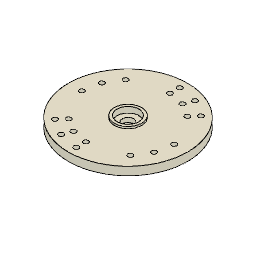
FT90R (Assembly) (Autodesk Fusion 360 archive; units mm, degrees)
design "Disc Servo Attachment"
Autodesk Fusion 360 part; units mm, degrees
sketch "Sketch1" plane through (0, 0, 0) normal (0, 1, 0) x (1, 0, 0)
  circle A0 centre (0, 0) radius 3.4163
  circle A1 centre (0, 0) radius 2.3241
  dimension "d1" = 6.8326
  dimension "d2" = 4.6482
  constraint coincident A0.centre A1.centre
  constraint concentric A0 A1
  measures "d1" diameter of A0
  measures "d2" diameter of A1
extrude "Extrude1" add sketch "Sketch1" along normal blind 2.3368 makes body 1
sketch "Sketch2" plane through (0, 2.3368, 0) normal (0, 1, 0) x (-1, 0, 0)
  circle A0 centre (0, 0) radius 2.3241
  circle A1 centre (0, 0) radius 3.4163
  circle A2 centre (0, 0) radius 11.8872
  circle A3 centre (0, 0) radius 1.1303
  dimension "d5" = 23.7744
  dimension "d6" = 2.2606
  constraint coincident A0.centre A1.centre
  constraint concentric A2 A3
  measures "d5" diameter of A2
  measures "d6" diameter of A3
extrude "Extrude2" add sketch "Sketch2" along normal blind 1.651 separate body contours A0 | A1 | A2 makes body 2
sketch "Sketch3" plane through (0, 3.9878, 0) normal (0, 1, 0) x (-1, 0, 0)
  circle A0 centre (0, 0) radius 1.1303
  circle A1 centre (0, 0) radius 11.8872
  circle A2 centre (0, 0) radius 2.7178
  circle A3 centre (0, 0) radius 2.1844
  dimension "d9" = 5.4356
  dimension "d10" = 4.3688
  constraint concentric A0 A2
  constraint coincident A0.centre A1.centre
  measures "d9" diameter of A2
  measures "d10" diameter of A3
extrude "Extrude3" add sketch "Sketch3" along normal blind 0.381 contours A2 bodies 2
sketch "Sketch4" plane through (0, 3.9878, 0) normal (0, 1, 0) x (-1, 0, 0)
  circle A0 centre (0, 0) radius 11.8872
  circle A1 centre (0, 0) radius 2.7178
  circle A2 centre (0, 0) radius 10.2872 construction
  circle A3 centre (0, 0) radius 9.2202 construction
  circle A4 centre (0, 0) radius 8.382 construction
  line L0 (0, 2.7178) -> (0, -10.795) construction
  circle A5 centre (-0.0124, -10.2872) radius 0.508
  circle A6 centre (0, -8.382) radius 0.508
  circle A7 centre (0, 0) radius 11.8872 construction
  line L1 (0, -10.795) -> (0, -11.8872) construction
  line L2 (0, -11.8872) -> (0, -8.89) construction
  circle A8 centre (-3.0695, -7.7998) radius 0.508
  circle A9 centre (-3.7556, -9.5771) radius 0.508
  circle A10 centre (-5.6936, -6.1515) radius 0.508
  circle A11 centre (-6.9837, -7.5534) radius 0.508
  line L3 (0.4991, -8.4767) -> (-3.5686, -7.7051) construction
  line L4 (0.4867, -10.3818) -> (-4.2547, -9.4824) construction
  line L5 (-2.6393, -8.07) -> (-6.1237, -5.8813) construction
  line L6 (-3.3252, -9.8469) -> (-7.4141, -7.2835) construction
  line L7 (0, 0) -> (-11.8872, 0) construction
  circle A12 centre (-9.2202, 0) radius 0.508
  line L8 (-11.8872, 0) -> (-9.7282, 0) construction
  circle A13 centre (-8.5826, 3.3692) radius 0.508
  circle A14 centre (-6.7579, 6.2724) radius 0.508
  line L9 (-9.3147, -0.4991) -> (-8.4881, 3.8683) construction
  line L10 (-8.8529, 2.9391) -> (-6.4876, 6.7025) construction
  circle A15 centre (0.0124, 10.2872) radius 0.508
  circle A16 centre (0, 8.382) radius 0.508
  circle A17 centre (3.7556, 9.5771) radius 0.508
  circle A18 centre (3.0695, 7.7998) radius 0.508
  circle A19 centre (6.9837, 7.5534) radius 0.508
  circle A20 centre (5.6936, 6.1515) radius 0.508
  circle A21 centre (9.2202, 0) radius 0.508
  circle A22 centre (8.5826, -3.3692) radius 0.508
  circle A23 centre (6.7579, -6.2724) radius 0.508
  dimension "d13" = 1.016
  dimension "d14" = 1.016
  dimension "d16" = 1.0922
  dimension "d17" = 2.9972
  dimension "d18" = 1.016
  dimension "d19" = 1.016
  dimension "d20" = 1.016
  dimension "d21" = 1.016
  dimension "d22" = 4.1402
  dimension "d23" = 4.826
  dimension "d24" = 4.1148
  dimension "d25" = 4.826
  dimension "d26" = 1.016
  dimension "d27" = 2.159
  dimension "d28" = 1.016
  dimension "d29" = 1.016
  dimension "d30" = 4.445
  dimension "d31" = 4.445
  dimension "d32" = 1.016
  dimension "d33" = 1.016
  dimension "d34" = 1.016
  dimension "d35" = 1.016
  dimension "d36" = 1.016
  dimension "d37" = 1.016
  dimension "d38" = 1.016
  dimension "d39" = 1.016
  dimension "d40" = 1.016
  constraint concentric A0 A2
  constraint concentric A0 A3
  constraint coincident A0.centre A1.centre
  constraint vertical L0
  constraint coincident A4 A6.centre
  constraint coincident L0 A6.centre
  constraint coincident A1 L0.start
  constraint concentric A4 A7
  constraint equal A0 A7
  constraint coincident A5 L0.end
  constraint coincident A7 L1.end
  constraint parallel L0 L1
  constraint coincident L0 L2.end
  constraint coincident A6 L2.end
  constraint coincident A2 A5.centre
  constraint coincident A4 A8.centre
  constraint coincident A2 A9.centre
  constraint coincident A4 A10.centre
  constraint coincident A2 A11.centre
  constraint coincident A6 L3.start
  constraint coincident A8 L3.end
  constraint coincident A5 L4.start
  constraint coincident A9 L4.end
  constraint parallel L3 L4
  constraint coincident A6.centre L3
  constraint coincident A8.centre L3
  constraint coincident A5.centre L4
  constraint coincident A9.centre L4
  constraint coincident A8 L5.start
  constraint coincident A10 L5.end
  constraint coincident A9 L6.start
  constraint coincident A11 L6.end
  constraint coincident A8.centre L5
  constraint coincident A10.centre L5
  constraint coincident A9.centre L6
  constraint coincident A11.centre L6
  constraint coincident A7 L7.end
  constraint perpendicular L0 L7
  constraint coincident A3 A12.centre
  constraint coincident L7 A12.centre
  constraint coincident A12 L8.end
  constraint coincident L7 L8.end
  constraint coincident A3 A13.centre
  constraint coincident A3 A14.centre
  constraint coincident A12 L9.start
  constraint coincident A13 L9.end
  constraint coincident A13 L10.start
  constraint coincident A14 L10.end
  constraint coincident A12.centre L9
  constraint coincident A13.centre L9
  constraint coincident A13.centre L10
  constraint coincident A14.centre L10
  constraint coincident A0.centre L0
  measures "d13" diameter of A5
  measures "d14" diameter of A6
  measures "d16" distance of L0.end L1.end
  measures "d17" distance of L1.end L2.end
  measures "d18" diameter of A8
  measures "d19" diameter of A9
  measures "d20" diameter of A10
  measures "d21" diameter of A11
  measures "d22" distance of L3.start L3.end
  measures "d23" distance of L4.start L4.end
  measures "d24" distance of L5.start L5.end
  measures "d25" distance of L6.start L6.end
  measures "d26" diameter of A12
  measures "d27" distance of L7.end L8.end
  measures "d28" diameter of A13
  measures "d29" diameter of A14
  measures "d30" distance of L9.start L9.end
  measures "d31" distance of L10.start L10.end
  measures "d32" diameter of A15
  measures "d33" diameter of A16
  measures "d34" diameter of A18
  measures "d35" diameter of A17
  measures "d36" diameter of A20
  measures "d37" diameter of A19
  measures "d38" diameter of A21
  measures "d39" diameter of A22
  measures "d40" diameter of A23
hole "Hole1" at (0.0124, 3.9878, -10.2872) at (0, 3.9878, -8.382) at (3.7556, 3.9878, -9.5771) at (3.0695, 3.9878, -7.7998) at (6.9837, 3.9878, -7.5534) at (5.6936, 3.9878, -6.1515) at (9.2202, 3.9878, 0) at (8.5826, 3.9878, 3.3692) at (6.7579, 3.9878, 6.2724) at (-0.0124, 3.9878, 10.2872) at (0, 3.9878, 8.382) at (-3.0695, 3.9878, 7.7998) at (-3.7556, 3.9878, 9.5771) at (-6.9837, 3.9878, 7.5534) at (-5.6936, 3.9878, 6.1515) at (-9.2202, 3.9878, 0) at (-8.5826, 3.9878, -3.3692) at (-6.7579, 3.9878, -6.2724) direction (0, -1, 0) diameter 1 end through all bodies 2
extrude "Extrude4" cut 1 faces at (-1.8207, 3.9878, -0.1647) along direction (0, -1, 0) blind 1.143 from surface at -0.381 on bodies 2 bodies 2

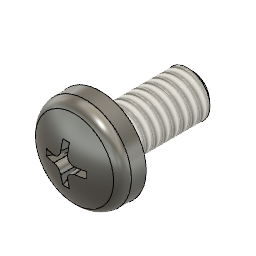
design "Pan Head Screw UNI EN ISO 7045 - M2 x 4 - H Steel 4.6 Plain"
description: Pan Head Screw UNI EN ISO 7045 - M2 x 4 - H
part number: UNI EN ISO 7045 - M2 x 4 - H Steel 4.6 Plain
Autodesk Fusion 360 part; units mm, degrees
sketch "Sketch1" plane through (0, 0, 0) normal (0, 1, 0) x (1, 0, 0)
  line L0 (-1, 0.8) -> (-1, 4)
  line L1 (-1, 4) -> (0, 4)
  line L2 (0, 4) -> (0, -1.6)
  line L3 (-0.8917, 0) -> (-2, 0)
  arc A0 (-1.9678, -0.9235) -> (0, -1.6) centre (0, 1.6) ccw
  line L4 (-1, 0.8) -> (-0.8917, 0.5678)
  line L5 (-0.8917, 0.5678) -> (-0.8917, 0)
  line L6 (-2, 0) -> (-1.9678, -0.9235)
  dimension "d9" = 2
  dimension "d66" = 4
  dimension "d75" = 1.7835
  dimension "d77" = 0.8
  dimension "d78" = 155
  dimension "d103" = 2
  dimension "d111" = 1.6
  dimension "d112" = 4
  constraint perpendicular L0 L1
  constraint collinear origin L2.end L1.end
  constraint perpendicular L0 L3
  constraint coincident origin L3
  constraint vertical L0
  constraint vertical L2
  constraint coincident L2 A0.centre
  constraint perpendicular L3 L5
  constraint coincident L3.start L5.end
  measures "d77" distance of L3 L0.start
  measures "d78" angle of L0 L4
  measures "d103" angle of L2 L6
  measures "d111" distance of L2.end L3
  measures "d112" distance of origin L1
revolve "Revolve1" add sketch "Sketch1" angle 360 about axis through (0, 0, -4) along (0, 0, 1) makes body 1
ref_plane "WorkPlane1" through (0, 0, 1.6) normal (0, 0, 1) x (1, 0, 0)
sketch "Sketch2" plane through (0, 0, 1.6) normal (0, 0, 1) x (1, 0, 0)
  line L0 (-0.15, 0.15) -> (-0.95, 0.15)
  line L1 (-0.15, -0.15) -> (-0.95, -0.15)
  line L2 (-0.95, 0.15) -> (-0.95, -0.15)
  line L3 (-0.15, -0.15) -> (-0.15, -0.95)
  line L4 (-0.15, -0.95) -> (0.15, -0.95)
  line L5 (0.15, -0.15) -> (0.15, -0.95)
  line L6 (0.15, -0.15) -> (0.95, -0.15)
  line L7 (0.95, -0.15) -> (0.95, 0.15)
  line L8 (0.15, 0.15) -> (0.95, 0.15)
  line L9 (0.15, 0.15) -> (0.15, 0.95)
  line L10 (0.15, 0.95) -> (-0.15, 0.95)
  line L11 (-0.15, 0.15) -> (-0.15, 0.95)
  dimension "d105" = 0.3
  dimension "d107" = 360
  dimension "d108" = 1.9
  constraint perpendicular L1 L2
  constraint vertical L0.start L1.start
  constraint horizontal L1
  constraint coincident L8.start L9.start
  measures "d105" distance of L0 L1
  measures "d108" distance of L2 L7
extrude "Extrude1" add sketch "Sketch2" against normal blind 1.2 draft -4 separate body makes body 2
draft "Draft1" angle -30 neutral plane through (0, 0, 1.6) pull (0, 0, 1) 4 faces at (-0.922, -0.022, 1.2) (-0.022, -0.922, 1.2) (0.922, -0.022, 1.2) (0.022, 0.922, 1.2) on bodies 2
fillet "Fillet3" radius 0.3 4 edges at (0.108, 0.108, 1) (-0.108, 0.108, 1) (0.108, -0.108, 1) (-0.108, -0.108, 1) on bodies 2
combine "Combine1" operation cut target body 1 tool bodies 2
fillet "Fillet4" radius 0.6 1 edges at (-1.8346, 0.7116, 0.9235) on bodies 1
thread "Thread1" "ISO Metric profile 2.0 M2x0.4 M2x0.4 6g" major diameter 1.9335 minor diameter 1.478 pitch 0.4 angle 60 resizes the face on face at (-0.9988, 0.0498, -1.8667) on bodies 1
fillet "Fillet5" radius 0.2 1 edges at (-0.8314, 0.3225, 0) on bodies 1
sketch "Sketch5" plane through (0, 0, 0) normal (0, 1, 0) x (1, 0, 0)
  line L0 (-1.02, 4) -> (-1.02, 3.7546)
  line L1 (-1.02, 3.7546) -> (-0.7546, 4)
  line L2 (0, 4) -> (0, -1.6)
  line L3 (-1.02, 4) -> (0, 4)
  dimension "d114" = 0.2454
  dimension "d115" = 1.02
  dimension "d116" = 0.2654
  constraint coincident L2.start L3.end
  constraint perpendicular L2 L3
  constraint coincident L1.end L3
  constraint perpendicular L0 L3
  measures "d114" distance of L0.end L3
  measures "d115" distance of L0 L2.start
  measures "d116" distance of L0 L1.end
revolve "Revolve2" cut sketch "Sketch5" angle 360 about axis through (0, 0, -4) along (0, 0, 1) bodies 1
equation "d9 = adsk_nomdia"
equation "adsk_nomlen = 4.00 mm"
equation "adsk_headh = 1.60 mm"
equation "adsk_headdia = 4.00 mm"
equation "adsk_nomdia = 2.00 mm"
equation "adsk_phildia = 1.90 mm"
equation "d31 = -adsk_phildepth"
equation "adsk_philwidth = 0.30 mm"
equation "adsk_phildepth = 1.20 mm"
equation "d66 = adsk_headdia"
equation "d71 = adsk_headh"
equation "adsk_thrlen = 3.20 mm"
equation "d75 = adsk_shnkdia"
equation "adsk_shnkdia = 1.78349 mm"
equation "d77 = adsk_nomlen - adsk_thrlen"
equation "adsk_endpointdia = 1.50924 mm"
equation "adsk_startlen = 0.24538 mm"
equation "adsk_ovalrad = 3.20 mm"
equation "adsk_headtoprad = adsk_nomdia * 0.3"
equation "adsk_midfillet = adsk_nomdia * 0.1"
equation "d98 = adsk_midfillet"
equation "adsk_headang = 2.00 deg"
equation "d102 = adsk_headtoprad"
equation "d103 = adsk_headang"
equation "d105 = adsk_philwidth"
equation "d108 = adsk_phildia"
equation "d110 = adsk_philwidth"
equation "d111 = adsk_headh"
equation "d112 = adsk_nomlen"
equation "d113 = ( adsk_nomlen + adsk_headh ) - ( adsk_ovalrad )"
equation "d114 = adsk_startlen"
equation "d115 = adsk_nomdia * 0.51"
equation "d116 = ( adsk_nomdia * 0.51 ) - ( adsk_endpointdia / 2 )"

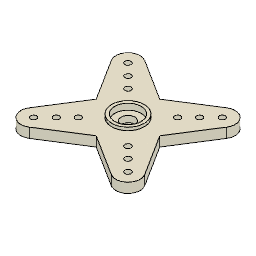
design "Square Servo Attachment"
Autodesk Fusion 360 part; units mm, degrees
sketch "Sketch1" plane through (0, 0, 0) normal (0, 1, 0) x (1, 0, 0)
  circle A0 centre (0, 0) radius 3.3909
  circle A1 centre (0, 0) radius 2.3368
  dimension "d1" = 6.7818
  dimension "d2" = 4.6736
  constraint coincident A0.centre A1.centre
  measures "d1" diameter of A0
  measures "d2" diameter of A1
extrude "Extrude1" add sketch "Sketch1" along normal blind 1.9304
sketch "Sketch2" plane through (0, 1.9304, 0) normal (0, 1, 0) x (-1, 0, 0)
  circle A0 centre (0, 0) radius 2.3368
  circle A1 centre (0, 0) radius 3.3909
  line L0 (-10.0076, 10.0076) -> (10.0076, 10.0076) construction
  line L1 (10.0076, 10.0076) -> (10.0076, -10.0076) construction
  line L2 (10.0076, -10.0076) -> (-10.0076, -10.0076) construction
  line L3 (-10.0076, -10.0076) -> (-10.0076, 10.0076) construction
  line L4 (-10.0076, 10.0076) -> (10.0076, -10.0076) construction
  line L5 (10.0076, 10.0076) -> (-10.0076, -10.0076) construction
  circle A2 centre (7.9709, -7.9709) radius 2.0367 construction
  circle A3 centre (-7.9709, -7.9709) radius 2.0367 construction
  circle A4 centre (-7.9709, 7.9709) radius 2.0367 construction
  circle A5 centre (7.9709, 7.9709) radius 2.0367 construction
  circle A6 centre (0, 0) radius 5.334 construction
  circle A7 centre (7.9709, -7.9709) radius 0.5
  circle A8 centre (-7.9709, -7.9709) radius 0.5
  circle A9 centre (7.9709, 7.9709) radius 0.5
  circle A10 centre (-7.9709, 7.9709) radius 0.5
  line L6 (8.4709, -7.9709) -> (-8.4709, -7.9709) construction
  line L7 (0, -5.334) -> (0, 5.334) construction
  line L8 (5.334, 0) -> (-5.334, 0) construction
  line L9 (9.4111, -6.5307) -> (6.5307, -9.4111) construction
  line L10 (-6.5307, -9.4111) -> (-9.4111, -6.5307) construction
  line L11 (-9.4111, 6.5307) -> (-6.5307, 9.4111) construction
  line L12 (9.4111, 6.5307) -> (6.5307, 9.4111) construction
  line L13 (5.334, 0) -> (9.6916, -6.8813)
  line L14 (5.334, 0) -> (9.6916, 6.8813)
  line L15 (0, 5.334) -> (6.8813, 9.6916)
  line L16 (0, 5.334) -> (-6.8813, 9.6916)
  line L17 (-5.334, 0) -> (-9.6916, 6.8813)
  line L18 (-5.334, 0) -> (-9.6916, -6.8813)
  line L19 (0, -5.334) -> (-6.8813, -9.6916)
  line L20 (0, -5.334) -> (6.8813, -9.6916)
  arc A11 (6.8813, -9.6916) -> (9.6916, -6.8813) centre (7.9709, -7.9709) ccw
  arc A12 (-9.6916, -6.8813) -> (-6.8813, -9.6916) centre (-7.9709, -7.9709) ccw
  arc A13 (-6.8813, 9.6916) -> (-9.6916, 6.8813) centre (-7.9709, 7.9709) ccw
  arc A14 (9.6916, 6.8813) -> (6.8813, 9.6916) centre (7.9709, 7.9709) ccw
  circle A15 centre (0, 0) radius 1.143
  dimension "d5" = 20.0152
  dimension "d6" = 20.0152
  dimension "d7" = 10.668
  dimension "d8" = 1
  dimension "d9" = 16.9418
  dimension "d10" = 2.286
  constraint horizontal L0
  constraint perpendicular L0 L1
  constraint parallel L0 L2
  constraint parallel L1 L3
  constraint coincident L4 A0.centre
  constraint coincident L5 A0.centre
  constraint coincident A0.centre A1.centre
  constraint coincident L4 A2.centre
  constraint coincident L5 A3.centre
  constraint coincident L4 A4.centre
  constraint coincident L5 A5.centre
  constraint tangent L2 A2
  constraint tangent L2 A3
  constraint tangent L3 A4
  constraint tangent L0 A5
  constraint equal A2 A3
  constraint equal A2 A4
  constraint equal A2 A5
  constraint concentric A2 A7
  constraint concentric A3 A8
  constraint concentric A5 A9
  constraint concentric A4 A10
  constraint equal A7 A8
  constraint equal A7 A9
  constraint equal A7 A10
  constraint coincident A7 L6.start
  constraint coincident A8 L6.end
  constraint coincident A2.centre L6
  constraint coincident A3.centre L6
  constraint coincident A6 L7.start
  constraint coincident A6 L7.end
  constraint coincident A0.centre L7
  constraint vertical L7
  constraint coincident A6 L8.start
  constraint coincident A6 L8.end
  constraint coincident A0.centre L8
  constraint horizontal L8
  constraint coincident A2 L9.start
  constraint coincident A2 L9.end
  constraint coincident A3 L10.start
  constraint coincident A3 L10.end
  constraint coincident A4 L11.start
  constraint coincident A4 L11.end
  constraint coincident A5 L12.start
  constraint coincident A5 L12.end
  constraint perpendicular L11 L12
  constraint coincident A2.centre L9
  constraint coincident A3.centre L10
  constraint coincident A4.centre L11
  constraint coincident A5.centre L12
  constraint perpendicular L4 L9
  constraint perpendicular L5 L10
  constraint perpendicular L4 L11
  constraint coincident A2 L13.end
  constraint coincident A5 L14.end
  constraint tangent A5 L14
  constraint coincident A5 L15.end
  constraint tangent A5 L15
  constraint coincident A4 L16.end
  constraint coincident A4 L17.end
  constraint tangent A4 L17
  constraint coincident A3 L18.end
  constraint coincident A3 L19.end
  constraint tangent A3 L19
  constraint coincident A2 L20.end
  constraint tangent A2 L13
  constraint tangent A2 L20
  constraint tangent A3 L18
  constraint tangent A4 L16
  constraint tangent L20 A11
  constraint tangent L18 A12
  constraint tangent L16 A13
  constraint tangent L15 A14
  measures "d5" distance of L1.end L2.end
  measures "d6" distance of L0.end L1.end
  measures "d7" diameter of A6
  measures "d8" diameter of A7
  measures "d9" distance of L6.start L6.end
  measures "d10" diameter of A15
extrude "Extrude2" add sketch "Sketch2" along normal blind 1.651 contours A0 | A1 | A7 | A8 | A9 | A10 | L13 L14 L15 L16 L17 L18 L19 L20 A11 A12 A13 A14
sketch "Sketch3" plane through (0, 3.5814, 0) normal (0, 1, 0) x (-1, 0, 0)
  circle A0 centre (0, 0) radius 1.143
  line L0 (5.334, 0) -> (9.6916, 6.8813)
  arc A1 (9.6916, 6.8813) -> (6.8813, 9.6916) centre (7.9709, 7.9709) ccw
  line L1 (6.8813, 9.6916) -> (0, 5.334)
  line L2 (0, 5.334) -> (-6.8813, 9.6916)
  arc A2 (-6.8813, 9.6916) -> (-9.6916, 6.8813) centre (-7.9709, 7.9709) ccw
  line L3 (-9.6916, 6.8813) -> (-5.334, 0)
  line L4 (-5.334, 0) -> (-9.6916, -6.8813)
  arc A3 (-9.6916, -6.8813) -> (-6.8813, -9.6916) centre (-7.9709, -7.9709) ccw
  line L5 (-6.8813, -9.6916) -> (0, -5.334)
  line L6 (0, -5.334) -> (6.8813, -9.6916)
  arc A4 (6.8813, -9.6916) -> (9.6916, -6.8813) centre (7.9709, -7.9709) ccw
  line L7 (9.6916, -6.8813) -> (5.334, 0)
  line L8 (-10.0076, 10.0076) -> (10.0076, 10.0076) construction
  line L9 (10.0076, 10.0076) -> (10.0076, -10.0076) construction
  line L10 (10.0076, -10.0076) -> (-10.0076, -10.0076) construction
  line L11 (-10.0076, -10.0076) -> (-10.0076, 10.0076) construction
  line L12 (-10.0076, 10.0076) -> (10.0076, -10.0076) construction
  line L13 (10.0076, 10.0076) -> (-10.0076, -10.0076) construction
  line L14 (8.2888, -8.2888) -> (-8.2888, 8.2888) construction
  line L15 (-8.2888, -8.2888) -> (8.2888, 8.2888) construction
  line L16 (-8.4455, 8.4455) -> (8.4455, 8.4455) construction
  line L17 (8.4455, 8.4455) -> (8.4455, -8.4455) construction
  line L18 (8.4455, -8.4455) -> (-8.4455, -8.4455) construction
  line L19 (-8.4455, -8.4455) -> (-8.4455, 8.4455) construction
  line L20 (-8.4455, 8.4455) -> (8.4455, -8.4455) construction
  line L21 (8.4455, 8.4455) -> (-8.4455, -8.4455) construction
  circle A5 centre (7.9104, -7.9104) radius 0.5351
  circle A6 centre (-7.9104, -7.9104) radius 0.5351
  circle A7 centre (-7.9104, 7.9104) radius 0.5351
  circle A8 centre (7.9104, 7.9104) radius 0.5351
  line L22 (-6.376, 6.376) -> (6.376, 6.376) construction
  line L23 (6.376, 6.376) -> (6.376, -6.376) construction
  line L24 (6.376, -6.376) -> (-6.376, -6.376) construction
  line L25 (-6.376, -6.376) -> (-6.376, 6.376) construction
  line L26 (-6.376, 6.376) -> (6.376, -6.376) construction
  line L27 (6.376, 6.376) -> (-6.376, -6.376) construction
  line L28 (-6.5278, 6.5278) -> (6.5278, 6.5278) construction
  line L29 (6.5278, 6.5278) -> (6.5278, -6.5278) construction
  line L30 (6.5278, -6.5278) -> (-6.5278, -6.5278) construction
  line L31 (-6.5278, -6.5278) -> (-6.5278, 6.5278) construction
  line L32 (-6.5278, 6.5278) -> (6.5278, -6.5278) construction
  line L33 (6.5278, 6.5278) -> (-6.5278, -6.5278) construction
  circle A9 centre (6.0095, -6.0095) radius 0.5183
  circle A10 centre (-6.0095, -6.0095) radius 0.5183
  circle A11 centre (-6.0095, 6.0095) radius 0.5183
  circle A12 centre (6.0095, 6.0095) radius 0.5183
  line L34 (-4.826, -4.826) -> (4.826, -4.826) construction
  line L35 (4.826, -4.826) -> (4.826, 4.826) construction
  line L36 (4.826, 4.826) -> (-4.826, 4.826) construction
  line L37 (-4.826, 4.826) -> (-4.826, -4.826) construction
  line L38 (-4.826, -4.826) -> (4.826, 4.826) construction
  line L39 (4.826, -4.826) -> (-4.826, 4.826) construction
  line L40 (-4.6338, -4.6338) -> (4.6338, -4.6338) construction
  line L41 (4.6338, -4.6338) -> (4.6338, 4.6338) construction
  line L42 (4.6338, 4.6338) -> (-4.6338, 4.6338) construction
  line L43 (-4.6338, 4.6338) -> (-4.6338, -4.6338) construction
  line L44 (-4.6338, -4.6338) -> (4.6338, 4.6338) construction
  line L45 (4.6338, -4.6338) -> (-4.6338, 4.6338) construction
  circle A13 centre (4.1698, -4.1698) radius 0.6562
  circle A14 centre (-4.1698, -4.1698) radius 0.6562
  circle A15 centre (-4.1698, 4.1698) radius 0.6562
  circle A16 centre (4.1698, 4.1698) radius 0.6562
  dimension "d13" = 23.4442
  dimension "d14" = 16.891
  dimension "d15" = 16.891
  dimension "d16" = 18.034
  dimension "d17" = 13.0556
  dimension "d18" = 13.1064
  dimension "d19" = 9.652
  constraint horizontal L8
  constraint perpendicular L8 L9
  constraint parallel L8 L10
  constraint parallel L9 L11
  constraint coincident L12 A0.centre
  constraint coincident L13 A0.centre
  constraint coincident A0.centre origin
  constraint tangent A4 L10
  constraint tangent A4 L9
  constraint coincident L12 L14.start
  constraint coincident L12 L14.end
  constraint midpoint A0.centre L14
  constraint coincident L13 L15.start
  constraint coincident L13 L15.end
  constraint midpoint A0.centre L15
  constraint equal L14 L15
  constraint horizontal L16
  constraint perpendicular L16 L17
  constraint parallel L16 L18
  constraint parallel L17 L19
  constraint coincident L20 A0.centre
  constraint coincident L21 A0.centre
  constraint coincident L12 A5.centre
  constraint coincident L15 A6.centre
  constraint coincident L14 A7.centre
  constraint coincident L21 A8.centre
  constraint coincident L14.start A5
  constraint coincident L15.start A6
  constraint coincident L14.end A7
  constraint coincident L15.end A8
  constraint tangent L18 A5
  constraint tangent L19 A6
  constraint tangent L19 A7
  constraint tangent L17 A8
  constraint horizontal L22
  constraint perpendicular L22 L23
  constraint parallel L22 L24
  constraint parallel L23 L25
  constraint coincident L26 A0.centre
  constraint coincident L27 A0.centre
  constraint coincident L20 L22.start
  constraint horizontal L28
  constraint perpendicular L28 L29
  constraint parallel L28 L30
  constraint parallel L29 L31
  constraint coincident L32 A0.centre
  constraint coincident L33 A0.centre
  constraint coincident L20 L28.start
  constraint coincident L14 A9.centre
  constraint coincident L33 A10.centre
  constraint coincident L32 A11.centre
  constraint coincident L33 A12.centre
  constraint coincident L23.end A9
  constraint coincident L24.end A10
  constraint coincident L22.start A11
  constraint coincident L22.end A12
  constraint tangent L30 A9
  constraint tangent L30 A10
  constraint tangent L28 A11
  constraint tangent L28 A12
  constraint horizontal L34
  constraint perpendicular L34 L35
  constraint parallel L34 L36
  constraint parallel L35 L37
  constraint coincident L38 A0.centre
  constraint coincident L39 A0.centre
  constraint coincident L15 L34.start
  constraint horizontal L40
  constraint perpendicular L40 L41
  constraint parallel L40 L42
  constraint parallel L41 L43
  constraint coincident L44 A0.centre
  constraint coincident L45 A0.centre
  constraint coincident L21 L40.start
  constraint coincident L39 A13.centre
  constraint coincident L13 A14.centre
  constraint coincident L26 A15.centre
  constraint coincident L15 A16.centre
  constraint coincident L40.end A13
  constraint coincident L40.start A14
  constraint coincident L42.end A15
  constraint coincident L41.end A16
  constraint tangent L34 A13
  constraint tangent L37 A14
  constraint tangent L37 A15
  constraint tangent L36 A16
  measures "d13" distance of L14.start L14.end
  measures "d14" distance of L17.end L18.end
  measures "d15" distance of L16.end L17.end
  measures "d16" distance of L22.start L23.end
  measures "d17" distance of L29.end L30.end
  measures "d18" distance of L40.end L42.end
  measures "d19" distance of L34.start L34.end
hole "Hole1" at (-7.9104, 3.5814, -7.9104) at (-6.0095, 3.5814, -6.0095) at (-4.1698, 3.5814, -4.1698) at (-7.9104, 3.5814, 7.9104) at (-6.0095, 3.5814, 6.0095) at (-4.1698, 3.5814, 4.1698) at (7.9104, 3.5814, 7.9104) at (6.0095, 3.5814, 6.0095) at (4.1698, 3.5814, 4.1698) at (7.9104, 3.5814, -7.9104) at (6.0095, 3.5814, -6.0095) at (4.1698, 3.5814, -4.1698) direction (0, -1, 0) diameter 1 end through all
sketch "Sketch4" plane through (0, 3.5814, 0) normal (0, 1, 0) x (-1, 0, 0)
  circle A0 centre (-6.0095, -6.0095) radius 0.5
  circle A1 centre (-4.1698, 4.1698) radius 0.5
  circle A2 centre (-7.9104, 7.9104) radius 0.5
  circle A3 centre (6.0095, 6.0095) radius 0.5
  circle A4 centre (4.1698, -4.1698) radius 0.5
  circle A5 centre (7.9104, -7.9104) radius 0.5
  circle A6 centre (6.0095, -6.0095) radius 0.5
  circle A7 centre (7.9104, 7.9104) radius 0.5
  circle A8 centre (4.1698, 4.1698) radius 0.5
  circle A9 centre (-6.0095, 6.0095) radius 0.5
  circle A10 centre (-7.9104, -7.9104) radius 0.5
  circle A11 centre (-4.1698, -4.1698) radius 0.5
  circle A12 centre (0, 0) radius 1.143
  line L0 (5.334, 0) -> (9.6916, 6.8813)
  arc A13 (9.6916, 6.8813) -> (6.8813, 9.6916) centre (7.9709, 7.9709) ccw
  line L1 (6.8813, 9.6916) -> (0, 5.334)
  line L2 (0, 5.334) -> (-6.8813, 9.6916)
  arc A14 (-6.8813, 9.6916) -> (-9.6916, 6.8813) centre (-7.9709, 7.9709) ccw
  line L3 (-9.6916, 6.8813) -> (-5.334, 0)
  line L4 (-5.334, 0) -> (-9.6916, -6.8813)
  arc A15 (-9.6916, -6.8813) -> (-6.8813, -9.6916) centre (-7.9709, -7.9709) ccw
  line L5 (-6.8813, -9.6916) -> (0, -5.334)
  line L6 (0, -5.334) -> (6.8813, -9.6916)
  arc A16 (6.8813, -9.6916) -> (9.6916, -6.8813) centre (7.9709, -7.9709) ccw
  line L7 (9.6916, -6.8813) -> (5.334, 0)
  circle A17 centre (0, 0) radius 2.7305
  circle A18 centre (0, 0) radius 2.2098
  dimension "d22" = 5.461
  dimension "d23" = 4.4196
  constraint coincident A12.centre A17.centre
  constraint concentric A12 A18
  measures "d22" diameter of A17
  measures "d23" diameter of A18
extrude "Extrude3" add sketch "Sketch4" along normal blind 0.508 contours A17
extrude "Extrude4" cut 1 faces at (-1.8417, 3.5814, -0.1666) along direction (0, -1, 0) blind 1.016 from surface at -0.508
extrude "Extrude5" cut 1 faces at (1.9259, 1.9304, 0.1729) along direction (0, 1, 0) blind 2.0066 from surface at -1.9304

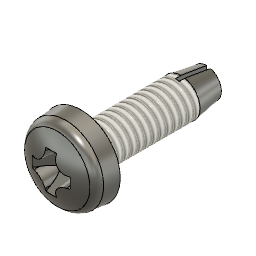
design "Type I Cross Recessed Pan Head Tapping Screw ASME B18.6.5M M2.5x0.45 x 8 Type D Steel Grade 2 Plain"
description: Type I Cross Recessed Pan Head Tapping Screw ASME B18.6.5M M2.5x0.45 x 8 Type D
part number: CRPHTS ASME B18.6.5M - M2.5x0.45 x 8  - D - I Steel Grade 2 Plain
Autodesk Fusion 360 part; units mm, degrees
sketch "Sketch1" plane through (0, 0, 0) normal (0, 1, 0) x (1, 0, 0)
  line L0 (-1.25, 0) -> (-1.25, 8)
  line L1 (-1.25, 8) -> (0, 8)
  line L2 (0, 8) -> (0, -2.1)
  line L3 (-1.25, 0) -> (-2.5, 0)
  arc A0 (-2.3853, -1.311) -> (0, -2.1) centre (0, 1.9) ccw
  line L4 (-2.5, 0) -> (-2.3853, -1.311)
  dimension "d9" = 2.5
  dimension "d66" = 5
  dimension "d127" = 5
  dimension "d129" = 2.1
  dimension "d138" = 8
  constraint perpendicular L0 L1
  constraint perpendicular L0 L3
  constraint coincident origin L3
  constraint vertical L0
  constraint vertical L2
  constraint coincident L2 A0.centre
  constraint coincident origin L2
  measures "d127" angle of L2 L4
  measures "d129" distance of L2.end L3
  measures "d138" distance of origin L1
revolve "Revolve1" add sketch "Sketch1" angle 360 about axis through (0, 0, -8) along (0, 0, 1) makes body 1
ref_plane "WorkPlane1" through (0, 0, 2.1) normal (0, 0, 1) x (1, 0, 0)
sketch "Sketch7" plane through (0, 0, 2.1) normal (0, 0, 1) x (1, 0, 0)
  line L0 (-0.35, -0.35) -> (-1.34, -0.35)
  line L1 (-1.34, 0.35) -> (-0.35, 0.35)
  line L2 (-1.34, -0.35) -> (-1.34, 0.35)
  line L3 (-0.35, -1.34) -> (-0.35, -0.35)
  line L4 (0.35, -1.34) -> (-0.35, -1.34)
  line L5 (0.35, -0.35) -> (0.35, -1.34)
  line L6 (1.34, -0.35) -> (0.35, -0.35)
  line L7 (1.34, 0.35) -> (1.34, -0.35)
  line L8 (0.35, 0.35) -> (1.34, 0.35)
  line L9 (0.35, 1.34) -> (0.35, 0.35)
  line L10 (-0.35, 1.34) -> (0.35, 1.34)
  line L11 (-0.35, 0.35) -> (-0.35, 1.34)
  dimension "d140" = 360
  dimension "d142" = 2.68
  dimension "d145" = 0.7
  constraint coincident L0.end L2.start
  constraint vertical L0.start L1.end
  constraint horizontal L1
  constraint coincident L1.end L11.start
  constraint perpendicular L7 L8
  measures "d142" distance of L2 L7.start
  measures "d145" distance of L0 L1
extrude "Extrude4" add sketch "Sketch7" against normal blind 1.53 draft -4 separate body makes body 2
draft "Draft2" angle -30 neutral plane through (0, 0, 2.1) pull (0, 0, 1) 4 faces at (-1.3043, 0.081, 1.59) (0.081, -1.3043, 1.59) (1.3043, 0.081, 1.59) (0.081, 1.3043, 1.59) on bodies 2
fillet "Fillet4" radius 0.7 4 edges at (-0.2965, 0.2965, 1.335) (-0.2965, -0.2965, 1.335) (0.2965, -0.2965, 1.335) (0.2965, 0.2965, 1.335) on bodies 2
combine "Combine1" operation cut target body 1 tool bodies 2
fillet "Fillet5" radius 0.7 1 edges at (-2.2239, 0.8626, 1.311) on bodies 1
thread "Thread1" "ANSI Metric M Profile 2.5 M2.5x0.45 M2.5x0.45 6g" major diameter 2.43 minor diameter 1.9165 pitch 0.45 angle 60 resizes the face on face at (-1.2438, 0.1245, -5.3333) on bodies 1
sketch "Sketch5" plane through (0, 0, 0) normal (0, 1, 0) x (1, 0, 0)
  line L0 (-1.275, 8) -> (-1.275, 6)
  line L1 (-1.275, 6) -> (-0.94, 8)
  line L2 (0, 8) -> (0, -2.1)
  line L3 (-1.275, 8) -> (0, 8)
  dimension "d131" = 2
  dimension "d132" = 1.275
  dimension "d133" = 0.335
  constraint coincident L2.start L3.end
  constraint perpendicular L2 L3
  constraint coincident L1.end L3
  constraint perpendicular L0 L3
  measures "d131" distance of L0.end L3
  measures "d132" distance of L0 L2.start
  measures "d133" distance of L0 L1.end
revolve "Revolve2" cut sketch "Sketch5" angle 360 about axis through (0, 0, -8) along (0, 0, 1) bodies 1
sketch "Sketch6" plane through (0, 0, -8) normal (0, 0, -1) x (-1, 0, 0)
  line L0 (0, 0) -> (-0.25, 0)
  line L1 (-0.25, 0) -> (-0.25, 2.5)
  line L2 (-0.25, 2.5) -> (0, 2.5)
  line L3 (0, 2.5) -> (0, 0)
  circle A0 centre (0, 0) radius 2.5
  dimension "d137" = 0.25
  constraint horizontal L0
  constraint vertical L1
  constraint coincident L0.start L3.end
  constraint horizontal L2
  constraint coincident L2.end A0
  measures "d137" distance of L1 L3
extrude "Extrude3" cut sketch "Sketch6" against normal blind 2 contours L0 L1 L2 L3 A0 bodies 1
equation "d9 = adsk_nomdia"
equation "adsk_nomlen = 8.00 mm"
equation "adsk_headh = 2.10 mm"
equation "adsk_headdia = 5.00 mm"
equation "adsk_nomdia = 2.50 mm"
equation "adsk_phildia = 2.68 mm"
equation "adsk_philwidth = 0.70 mm"
equation "adsk_phildepth = 1.53 mm"
equation "d66 = adsk_headdia"
equation "d71 = adsk_headh"
equation "adsk_startlen = 2.00 mm"
equation "adsk_endpointdia = 1.88 mm"
equation "d110 = -adsk_startlen"
equation "d114 = -adsk_phildepth"
equation "adsk_ovalrad = 4.00 mm"
equation "adsk_headtoprad = adsk_headh / 3"
equation "d125 = adsk_headtoprad"
equation "adsk_headang = 5 deg"
equation "d127 = adsk_headang"
equation "d129 = adsk_headh"
equation "d130 = ( adsk_nomlen + adsk_headh ) - ( adsk_ovalrad )"
equation "d131 = adsk_startlen"
equation "d132 = adsk_nomdia * 0.51"
equation "d133 = ( 0.51 * adsk_nomdia ) - ( adsk_endpointdia / 2 )"
equation "d137 = adsk_nomdia / 10"
equation "d138 = adsk_nomlen"
equation "d142 = adsk_phildia"
equation "d144 = adsk_philwidth"
equation "d145 = adsk_philwidth"
